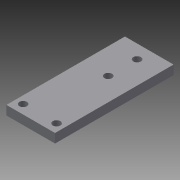
# Autodesk Inventor part: bart x endstop bracket plain switch v1
Saved by Autodesk Inventor 2014 SP1 (Build 180222100, 222)
## iProperties
Created: 2015-12-23
Part Number: bart x endstop bracket plain switch v1
Material: Generic
Document SubType Name: Modeling
Designer: Mon
Density: 1 g/cm^3
Appearance: Default
Author: Mon
Autodesk Inventor part; units mm, degrees
ref_plane "YZ Plane" through (0, 0, 0) normal (1, 0, 0) x (0, 1, 0)
ref_plane "XZ Plane" through (0, 0, 0) normal (0, 1, 0) x (-1, 0, 0)
ref_plane "XY Plane" through (0, 0, 0) normal (0, 0, 1) x (1, 0, 0)
sketch "Sketch1" plane through (0, 0, 0) normal (0, 0, 1) x (1, 0, 0)
  line L0 (0, 0) -> (16, 0)
  line L1 (16, 0) -> (16, 39)
  line L2 (16, 39) -> (0, 39)
  line L3 (0, 39) -> (0, 0)
  line L4 (8, 32.7385) -> (8, -1.6019) construction
  line L5 (8, 0) -> (8, 3) construction
  line L6 (8, 3) -> (-6.2893, 3) construction
  line L7 (-6.2893, 3) -> (30.6517, 3) construction
  line L8 (8, 3) -> (13.5, 3) construction
  line L9 (13.5, 3) -> (13.5, 7.8913) construction
  line L10 (13.5, 7.8913) -> (2.5, 7.8913) construction
  line L11 (2.5, 7.8913) -> (2.5, 1.5) construction
  circle A0 centre (2.5, 3) radius 1.25
  circle A1 centre (13.5, 3) radius 1.25
  line L12 (8, 0) -> (8, 25) construction
  line L13 (8, 25) -> (38.3893, 25) construction
  line L14 (38.3893, 25) -> (38.3893, 34.5) construction
  line L15 (38.3893, 34.5) -> (16, 34.5) construction
  line L16 (16, 34.5) -> (8.5, 34.5) construction
  line L17 (8.5, 34.5) -> (8.5, 22.056) construction
  circle A2 centre (8.5, 34.5) radius 1.25
  circle A3 centre (8.5, 25) radius 1.25
  dimension "d0" = 16
  dimension "d1" = 39
  dimension "d2" = 3
  dimension "d3" = 5.5
  dimension "d4" = 11
  dimension "d5" = 2.5
  dimension "d6" = 2.5
  dimension "d7" = 25
  dimension "d8" = 9.5
  dimension "d9" = 7.5
  dimension "d10" = 2.5
  dimension "d11" = 2.5
  constraints: 36 end point, 9 point on line, 7 perpendicular, 6 parallel, 4 centre point, 2 coincident, 1 collinear, 1 horizontal, 1 midpoint
  measures "d0" distance of L2.end L1.end
  measures "d1" distance of L1.end L0.end
  measures "d2" distance of L5.start L5.end
  measures "d3" distance of L5.end L8.end
  measures "d4" distance of L9.end L10.end
  measures "d5" diameter of A0
  measures "d6" diameter of A1
  measures "d7" distance of L5.start L12.end
  measures "d8" distance of L13.end L14.end
  measures "d9" distance of L15.end L16.end
  measures "d10" diameter of A2
  measures "d11" diameter of A3
extrude "Extrusion1" add sketch "Sketch1" along normal blind 3
body "Solid1"
